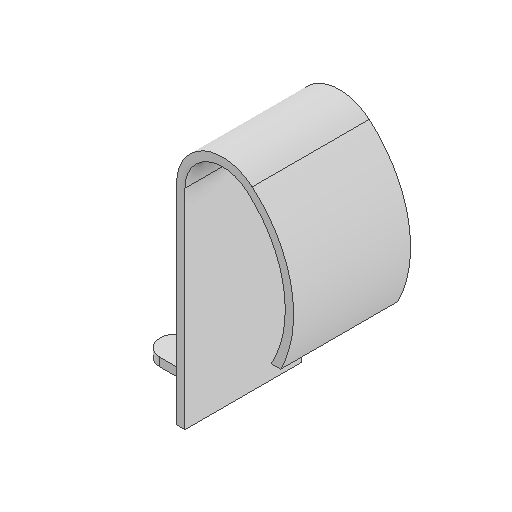
# Autodesk Inventor part: Holder_Metal
Saved by Autodesk Inventor 2025.2 (Build 292293000, 293)
## iProperties
Created: 2025-03-09
Part Number: Holder_Metal
Material: Generic
Document SubType Name: Modeling
Designer: ahorat
Density: 1 g/cm^3
Appearance: Default
Author: ahorat
Autodesk Inventor part; units mm, degrees
ref_plane "YZ Plane" through (0, 0, 0) normal (1, 0, 0) x (0, 1, 0)
ref_plane "XZ Plane" through (0, 0, 0) normal (0, 1, 0) x (-1, 0, 0)
ref_plane "XY Plane" through (0, 0, 0) normal (0, 0, 1) x (1, 0, 0)
sketch "Sketch1" plane through (0, 0, 0) normal (0, 0, 1) x (1, 0, 0)
  line L0 (0, 0) -> (0, 12.5096)
  arc A0 (4.5242, 14.5927) -> (0, 12.5096) centre (2.7416, 12.5096) ccw
  arc A1 (6.2274, 6) -> (4.5242, 14.5927) centre (-0.0774, 9.2154) ccw
  line L1 (6.2274, 6) -> (5.6605, 6)
  arc A2 (5.6605, 6) -> (4.1991, 14.2128) centre (-0.0774, 9.2154) ccw
  arc A3 (4.1991, 14.2128) -> (0.5, 12.5096) centre (2.7416, 12.5096) ccw
  line L2 (0.5, 12.5096) -> (0.5, 0)
  line L3 (0, 0) -> (0.5, 0)
  line L4 (7, 9.2154) -> (7, 0)
  point P0 (0.25, 0)
  point P1 (1.595, 15)
  point P2 (5.9439, 6)
  point P3 (6.8649, 10.5915)
  dimension "d0" = 0.5
  dimension "d1" = 15
  dimension "d2" = 6
  dimension "d4" = 7
  constraints: 11 point on circle, 10 end point, 5 tangent, 4 centre point, 3 vertical, 2 horizontal, 2 midpoint, 1 coincident, 1 concentric
  measures "d0" distance between parallel lines of L0 L2
  measures "d1" vertical distance of point (0.25, 0) point (1.595, 15)
  measures "d2" vertical distance of point (0.25, 0) point (5.944, 6)
  measures "d4" distance between parallel lines of L0 L4
extrude "Extrusion1" add sketch "Sketch1" along normal mid plane 7
sketch "Sketch2" plane through (0, 0, -3.5) normal (-1, 0, 0) x (0, 0, 1)
  line L0 (2.5, 0) -> (4.5, 0)
  line L1 (4.5, 0) -> (4.5, 0.5)
  line L2 (4.5, 0.5) -> (2.5, 0.5)
  line L3 (2.5, 0.5) -> (2.5, 0)
  line L4 (0, 0) -> (7, 0) projected
  point P0 (3.5, 0.5)
  point P1 (3.5, 0)
  dimension "d8" = 2
  constraints: 8 end point, 3 midpoint, 2 parallel, 1 horizontal, 1 perpendicular
  measures "d8" distance of L1.end L2.end
extrude "Extrusion2" add sketch "Sketch2" along normal blind 4.5
fillet "Fillet1" radius 1 2 edges at (-4.5, 0.25, 1) (-4.5, 0.25, -1)
body "Solid1"
